Autodesk Inventor part; units mm, degrees
(part 2 of 2)
  arc A140 (-25.4446, 74.7133) -> (-26.798, 74.2336) centre (-25.1834, 71.8276) ccw
  arc A141 (-26.798, 74.2336) -> (-27.2062, 73.5932) centre (-26.3001, 73.4659) ccw
  arc A142 (-21.4794, 73.1947) -> (-22.0085, 74.2336) centre (-22.7699, 73.1916) ccw
  circle A143 centre (-25.9605, 73.338) radius 0.5161
  line L109 (-27.2062, 73.5932) -> (-27.2062, 72.1245)
  line L110 (-27.2062, 72.1245) -> (-24.3395, 72.1245)
  line L111 (-24.3395, 71.7056) -> (-28.3839, 71.7056)
  line L112 (-24.3395, 72.1245) -> (-24.3395, 71.7056)
  line L113 (-21.4733, 70.5884) -> (-21.4794, 73.1947)
  arc A144 (-23.3243, 25.8454) -> (-25.4322, 25.8454) centre (-24.3782, 17.6506) ccw
  arc A145 (-25.4322, 25.8454) -> (-26.7856, 25.3656) centre (-25.171, 22.9597) ccw
  arc A146 (-21.9961, 25.3656) -> (-23.3243, 25.8454) centre (-23.7019, 22.7218) ccw
  arc A147 (-21.4671, 24.3267) -> (-21.9961, 25.3656) centre (-22.7575, 24.3237) ccw
  arc A148 (-26.7856, 25.3656) -> (-27.1938, 24.7252) centre (-26.2877, 24.5979) ccw
  circle A149 centre (-25.9607, 24.5305) radius 0.545
  line L114 (-27.1938, 24.7252) -> (-27.1938, 23.2566)
  line L115 (-27.1938, 23.2566) -> (-24.3272, 23.2566)
  line L116 (-24.3272, 23.2566) -> (-24.3272, 22.8376)
  line L117 (-21.461, 21.7204) -> (-21.4671, 24.3267)
  line L118 (-26.0801, 20.1743) -> (-23.0926, 20.1813)
  arc A150 (-22.5618, 19.8544) -> (-21.3196, 20.5365) centre (-22.5875, 21.3734) ccw
  arc A151 (-23.0926, 20.1813) -> (-21.461, 21.7204) centre (-22.9431, 21.6573) ccw
  line L119 (-22.5618, 19.8544) -> (-25.5493, 19.8474)
  line L120 (-21.0597, 22.9429) -> (-21.0597, 21.4689)
  arc A152 (-21.3196, 20.5365) -> (-21.0597, 21.4689) centre (-22.9439, 21.4916) ccw
  line L121 (-19.9288, 22.9429) -> (-21.0597, 22.9429)
  arc A153 (-18.7198, 21.9341) -> (-19.9288, 22.9429) centre (-20.2582, 21.3193) ccw
  arc A154 (-18.5273, 18.7011) -> (-18.7198, 21.9341) centre (-23.4893, 20.0279) ccw
  arc A155 (-20.2704, 17.1911) -> (-18.5273, 18.7011) centre (-20.3549, 19.0497) ccw
  arc A156 (-25.5493, 19.8474) -> (-27.181, 18.3083) centre (-25.6988, 18.3715) ccw
  arc A157 (-26.0801, 20.1743) -> (-27.3224, 19.4922) centre (-26.0545, 18.6554) ccw
  line L122 (-24.3272, 22.8376) -> (-28.3715, 22.8376)
  arc A158 (-27.3224, 19.4922) -> (-27.5822, 18.5598) centre (-25.698, 18.5371) ccw
  line L123 (-27.5822, 17.0858) -> (-27.5822, 18.5598)
  arc A159 (-28.3715, 22.8376) -> (-30.1146, 21.3277) centre (-28.287, 20.979) ccw
  line L124 (-28.7131, 17.0858) -> (-27.5822, 17.0858)
  arc A160 (-30.1146, 21.3277) -> (-29.9221, 18.0946) centre (-25.1526, 20.0009) ccw
  arc A161 (-29.9221, 18.0946) -> (-28.7131, 17.0858) centre (-28.3837, 18.7095) ccw
  arc A162 (-25.3176, 14.1834) -> (-23.2097, 14.1834) centre (-24.2637, 22.3782) ccw
  arc A163 (-26.6458, 14.6631) -> (-25.3176, 14.1834) centre (-24.94, 17.307) ccw
  arc A164 (-23.2097, 14.1834) -> (-21.8563, 14.6631) centre (-23.4709, 17.0691) ccw
  arc A165 (-21.8563, 14.6631) -> (-21.4481, 15.3035) centre (-22.3542, 15.4308) ccw
  arc A166 (-27.1749, 15.702) -> (-26.6458, 14.6631) centre (-25.8844, 15.705) ccw
  circle A167 centre (-22.6938, 15.5587) radius 0.5161
  line L125 (-21.4481, 15.3035) -> (-21.4481, 16.7721)
  line L126 (-21.4481, 16.7721) -> (-24.3148, 16.7721)
  line L127 (-24.3148, 17.1911) -> (-20.2704, 17.1911)
  line L128 (-24.3148, 16.7721) -> (-24.3148, 17.1911)
  line L129 (-27.181, 18.3083) -> (-27.1749, 15.702)
  arc A168 (-40.1766, 38.6055) -> (-38.0687, 38.6055) centre (-39.1227, 46.8003) ccw
  arc A169 (-38.0687, 38.6055) -> (-36.7153, 39.0853) centre (-38.3299, 41.4912) ccw
  arc A170 (-41.5048, 39.0853) -> (-40.1766, 38.6055) centre (-39.799, 41.7291) ccw
  arc A171 (-42.0338, 40.1242) -> (-41.5048, 39.0853) centre (-40.7434, 40.1272) ccw
  arc A172 (-36.7153, 39.0853) -> (-36.3071, 39.7256) centre (-37.2132, 39.853) ccw
  circle A173 centre (-37.5402, 39.9204) radius 0.545
  line L130 (-36.3071, 39.7256) -> (-36.3071, 41.1943)
  line L131 (-36.3071, 41.1943) -> (-39.1737, 41.1943)
  line L132 (-39.1737, 41.1943) -> (-39.1737, 41.6132)
  line L133 (-42.0399, 42.7305) -> (-42.0338, 40.1242)
  line L134 (-37.4208, 44.2766) -> (-40.4083, 44.2696)
  arc A174 (-40.9391, 44.5964) -> (-42.1813, 43.9143) centre (-40.9134, 43.0775) ccw
  arc A175 (-40.4083, 44.2696) -> (-42.0399, 42.7305) centre (-40.5578, 42.7936) ccw
  line L135 (-40.9391, 44.5964) -> (-37.9516, 44.6034)
  line L136 (-42.4412, 41.508) -> (-42.4412, 42.982)
  arc A176 (-42.1813, 43.9143) -> (-42.4412, 42.982) centre (-40.557, 42.9593) ccw
  line L137 (-43.5721, 41.508) -> (-42.4412, 41.508)
  arc A177 (-44.7811, 42.5167) -> (-43.5721, 41.508) centre (-43.2427, 43.1316) ccw
  arc A178 (-44.9736, 45.7498) -> (-44.7811, 42.5167) centre (-40.0116, 44.423) ccw
  arc A179 (-43.2305, 47.2598) -> (-44.9736, 45.7498) centre (-43.146, 45.4011) ccw
  arc A180 (-37.9516, 44.6034) -> (-36.3199, 46.1426) centre (-37.8021, 46.0794) ccw
  arc A181 (-37.4208, 44.2766) -> (-36.1785, 44.9587) centre (-37.4464, 45.7955) ccw
  line L138 (-39.1737, 41.6132) -> (-35.1294, 41.6132)
  arc A182 (-36.1785, 44.9587) -> (-35.9187, 45.891) centre (-37.8029, 45.9137) ccw
  line L139 (-35.9187, 47.365) -> (-35.9187, 45.891)
  arc A183 (-35.1294, 41.6132) -> (-33.3863, 43.1232) centre (-35.2139, 43.4719) ccw
  line L140 (-34.7877, 47.365) -> (-35.9187, 47.365)
  arc A184 (-33.3863, 43.1232) -> (-33.5788, 46.3563) centre (-38.3483, 44.45) ccw
  arc A185 (-33.5788, 46.3563) -> (-34.7877, 47.365) centre (-35.1172, 45.7414) ccw
  arc A186 (-38.1832, 50.2675) -> (-40.2912, 50.2675) centre (-39.2372, 42.0727) ccw
  arc A187 (-36.8551, 49.7878) -> (-38.1832, 50.2675) centre (-38.5609, 47.1439) ccw
  arc A188 (-40.2912, 50.2675) -> (-41.6446, 49.7878) centre (-40.03, 47.3818) ccw
  arc A189 (-41.6446, 49.7878) -> (-42.0528, 49.1474) centre (-41.1467, 49.02) ccw
  arc A190 (-36.326, 48.7488) -> (-36.8551, 49.7878) centre (-37.6165, 48.7458) ccw
  circle A191 centre (-40.8071, 48.8922) radius 0.5161
  line L141 (-42.0528, 49.1474) -> (-42.0528, 47.6787)
  line L142 (-42.0528, 47.6787) -> (-39.1861, 47.6787)
  line L143 (-39.1861, 47.2598) -> (-43.2305, 47.2598)
  line L144 (-39.1861, 47.6787) -> (-39.1861, 47.2598)
  line L145 (-36.3199, 46.1426) -> (-36.326, 48.7488)
  line L146 (-31.75, 88.9) -> (-31.75, 0) construction
  arc A192 (-25.3307, 38.6055) -> (-23.2228, 38.6055) centre (-24.2767, 46.8003) ccw
  arc A193 (-23.2228, 38.6055) -> (-21.8693, 39.0853) centre (-23.4839, 41.4912) ccw
  arc A194 (-20.2834, 41.6132) -> (-18.5403, 43.1232) centre (-20.3679, 43.4719) ccw
  arc A195 (-21.3326, 44.9587) -> (-21.0728, 45.891) centre (-22.9569, 45.9137) ccw
  arc A196 (-18.5403, 43.1232) -> (-18.7328, 46.3563) centre (-23.5023, 44.45) ccw
  arc A197 (-18.7328, 46.3563) -> (-19.9418, 47.365) centre (-20.2712, 45.7414) ccw
  line L147 (-19.9418, 47.365) -> (-21.0728, 47.365)
  line L148 (-21.0728, 47.365) -> (-21.0728, 45.891)
  line L149 (-22.5749, 44.2766) -> (-25.5624, 44.2696)
  line L150 (-26.0931, 44.5964) -> (-23.1056, 44.6034)
  line L151 (-24.3402, 47.6787) -> (-24.3402, 47.2598)
  line L152 (-24.3402, 47.2598) -> (-28.3846, 47.2598)
  line L153 (-21.474, 46.1426) -> (-21.4801, 48.7488)
  line L154 (-27.2069, 47.6787) -> (-24.3402, 47.6787)
  circle A198 centre (-25.9611, 48.8922) radius 0.5161
  line L155 (-27.2069, 49.1474) -> (-27.2069, 47.6787)
  arc A199 (-26.7987, 49.7878) -> (-27.2069, 49.1474) centre (-26.3007, 49.02) ccw
  arc A200 (-25.4452, 50.2675) -> (-26.7987, 49.7878) centre (-25.1841, 47.3818) ccw
  arc A201 (-23.3373, 50.2675) -> (-25.4452, 50.2675) centre (-24.3913, 42.0727) ccw
  arc A202 (-22.0092, 49.7878) -> (-23.3373, 50.2675) centre (-23.7149, 47.1439) ccw
  arc A203 (-21.4801, 48.7488) -> (-22.0092, 49.7878) centre (-22.7706, 48.7458) ccw
  arc A204 (-21.8693, 39.0853) -> (-21.4611, 39.7256) centre (-22.3673, 39.853) ccw
  circle A205 centre (-22.6942, 39.9204) radius 0.545
  line L156 (-21.4611, 39.7256) -> (-21.4611, 41.1943)
  line L157 (-21.4611, 41.1943) -> (-24.3278, 41.1943)
  line L158 (-24.3278, 41.6132) -> (-20.2834, 41.6132)
  line L159 (-24.3278, 41.1943) -> (-24.3278, 41.6132)
  arc A206 (-22.5749, 44.2766) -> (-21.3326, 44.9587) centre (-22.6005, 45.7955) ccw
  arc A207 (-23.1056, 44.6034) -> (-21.474, 46.1426) centre (-22.9562, 46.0794) ccw
  arc A208 (-26.6588, 39.0853) -> (-25.3307, 38.6055) centre (-24.9531, 41.7291) ccw
  arc A209 (-27.1879, 40.1242) -> (-26.6588, 39.0853) centre (-25.8974, 40.1272) ccw
  line L160 (-27.194, 42.7305) -> (-27.1879, 40.1242)
  arc A210 (-26.0931, 44.5964) -> (-27.3354, 43.9143) centre (-26.0675, 43.0775) ccw
  arc A211 (-25.5624, 44.2696) -> (-27.194, 42.7305) centre (-25.7118, 42.7936) ccw
  line L161 (-27.5952, 41.508) -> (-27.5952, 42.982)
  arc A212 (-27.3354, 43.9143) -> (-27.5952, 42.982) centre (-25.7111, 42.9593) ccw
  arc A213 (-28.3846, 47.2598) -> (-30.1277, 45.7498) centre (-28.3001, 45.4011) ccw
  line L162 (-28.7262, 41.508) -> (-27.5952, 41.508)
  arc A214 (-29.9351, 42.5167) -> (-28.7262, 41.508) centre (-28.3968, 43.1316) ccw
  arc A215 (-30.1277, 45.7498) -> (-29.9351, 42.5167) centre (-25.1657, 44.423) ccw
  line L163 (-39.1737, 68.8958) -> (-24.3278, 44.45) construction
  line L164 (-39.1737, 44.45) -> (-24.3272, 68.8958) construction
  arc A216 (-32.7536, 50.8283) -> (-30.6456, 50.8283) centre (-31.6996, 59.0231) ccw
  arc A217 (-30.6456, 50.8283) -> (-29.2922, 51.308) centre (-30.9068, 53.714) ccw
  arc A218 (-34.0817, 51.308) -> (-32.7536, 50.8283) centre (-32.3759, 53.9519) ccw
  arc A219 (-34.6108, 52.3469) -> (-34.0817, 51.308) centre (-33.3203, 52.3499) ccw
  arc A220 (-29.2922, 51.308) -> (-28.884, 51.9484) centre (-29.7901, 52.0757) ccw
  circle A221 centre (-30.1171, 52.1431) radius 0.545
  line L165 (-28.884, 51.9484) -> (-28.884, 53.417)
  line L166 (-28.884, 53.417) -> (-31.7507, 53.417)
  line L167 (-31.7507, 53.417) -> (-31.7507, 53.836)
  line L168 (-34.6169, 54.9532) -> (-34.6108, 52.3469)
  line L169 (-29.9978, 56.4993) -> (-32.9852, 56.4923)
  arc A222 (-33.516, 56.8192) -> (-34.7583, 56.1371) centre (-33.4904, 55.3003) ccw
  arc A223 (-32.9852, 56.4923) -> (-34.6169, 54.9532) centre (-33.1347, 55.0164) ccw
  line L170 (-33.516, 56.8192) -> (-30.5285, 56.8262)
  line L171 (-35.0181, 53.7307) -> (-35.0181, 55.2047)
  arc A224 (-34.7583, 56.1371) -> (-35.0181, 55.2047) centre (-33.1339, 55.182) ccw
  line L172 (-36.1491, 53.7307) -> (-35.0181, 53.7307)
  arc A225 (-37.358, 54.7395) -> (-36.1491, 53.7307) centre (-35.8197, 55.3544) ccw
  arc A226 (-37.5506, 57.9726) -> (-37.358, 54.7395) centre (-32.5885, 56.6458) ccw
  arc A227 (-35.8074, 59.4825) -> (-37.5506, 57.9726) centre (-35.7229, 57.6239) ccw
  arc A228 (-30.5285, 56.8262) -> (-28.8969, 58.3653) centre (-30.379, 58.3022) ccw
  arc A229 (-29.9978, 56.4993) -> (-28.7555, 57.1814) centre (-30.0234, 58.0183) ccw
  line L173 (-31.7507, 53.836) -> (-27.7063, 53.836)
  arc A230 (-28.7555, 57.1814) -> (-28.4957, 58.1138) centre (-30.3798, 58.1365) ccw
  line L174 (-28.4957, 59.5878) -> (-28.4957, 58.1138)
  arc A231 (-27.7063, 53.836) -> (-25.9632, 55.346) centre (-27.7908, 55.6946) ccw
  line L175 (-27.3647, 59.5878) -> (-28.4957, 59.5878)
  arc A232 (-25.9632, 55.346) -> (-26.1557, 58.579) centre (-30.9252, 56.6728) ccw
  arc A233 (-26.1557, 58.579) -> (-27.3647, 59.5878) centre (-27.6941, 57.9642) ccw
  arc A234 (-30.7602, 62.4903) -> (-32.8681, 62.4903) centre (-31.8141, 54.2955) ccw
  arc A235 (-29.4321, 62.0105) -> (-30.7602, 62.4903) centre (-31.1378, 59.3667) ccw
  arc A236 (-32.8681, 62.4903) -> (-34.2215, 62.0105) centre (-32.607, 59.6046) ccw
  arc A237 (-34.2215, 62.0105) -> (-34.6298, 61.3701) centre (-33.7236, 61.2428) ccw
  arc A238 (-28.903, 60.9716) -> (-29.4321, 62.0105) centre (-30.1934, 60.9686) ccw
  circle A239 centre (-33.384, 61.1149) radius 0.5161
  line L176 (-34.6298, 61.3701) -> (-34.6298, 59.9015)
  line L177 (-34.6298, 59.9015) -> (-31.7631, 59.9015)
  line L178 (-31.7631, 59.4825) -> (-35.8074, 59.4825)
  line L179 (-31.7631, 59.9015) -> (-31.7631, 59.4825)
  line L180 (-28.8969, 58.3653) -> (-28.903, 60.9716)
  line L181 (-50.4381, 84.1079) -> (-54.8347, 75.4711)
  line L182 (-54.8347, 75.4711) -> (-56.2838, 75.4711)
  line L183 (-56.2838, 75.4711) -> (-51.6402, 84.4373)
  line L184 (-51.6402, 84.4373) -> (-56.8849, 84.4373)
  line L185 (-56.8849, 84.4373) -> (-56.8849, 85.6311)
  line L186 (-56.8849, 85.6311) -> (-50.4381, 85.6311)
  line L187 (-50.4381, 85.6311) -> (-50.4381, 84.1079)
  line L188 (-13.0619, 5.1366) -> (-8.6653, 13.7735)
  line L189 (-8.6653, 13.7735) -> (-7.2162, 13.7735)
  line L190 (-7.2162, 13.7735) -> (-11.8598, 4.8073)
  line L191 (-11.8598, 4.8073) -> (-6.6151, 4.8073)
  line L192 (-6.6151, 4.8073) -> (-6.6151, 3.6135)
  line L193 (-6.6151, 3.6135) -> (-13.0619, 3.6135)
  line L194 (-13.0619, 3.6135) -> (-13.0619, 5.1366)
  line L195 (-50.4381, 84.1079) -> (-54.8347, 75.4711)
  line L196 (-54.8347, 75.4711) -> (-56.2838, 75.4711)
  line L197 (-56.2838, 75.4711) -> (-51.6402, 84.4373)
  line L198 (-51.6402, 84.4373) -> (-56.8849, 84.4373)
  line L199 (-56.8849, 84.4373) -> (-56.8849, 85.6311)
  line L200 (-56.8849, 85.6311) -> (-50.4381, 85.6311)
  line L201 (-50.4381, 85.6311) -> (-50.4381, 84.1079)
  line L202 (-13.0619, 5.1366) -> (-8.6653, 13.7735)
  line L203 (-8.6653, 13.7735) -> (-7.2162, 13.7735)
  line L204 (-7.2162, 13.7735) -> (-11.8598, 4.8073)
  line L205 (-11.8598, 4.8073) -> (-6.6151, 4.8073)
  line L206 (-6.6151, 4.8073) -> (-6.6151, 3.6135)
  line L207 (-6.6151, 3.6135) -> (-13.0619, 3.6135)
  line L208 (-13.0619, 3.6135) -> (-13.0619, 5.1366)
  point P0 (-39.1737, 20.0009)
  point P1 (-53.7479, 68.8958)
  point P2 (-9.7521, 20.0042)
  point P3 (-13.4723, 102.9238)
  point P4 (-39.1737, 20.0009)
  point P5 (-53.7479, 68.8958)
  point P6 (-9.7521, 20.0042)
  point P7 (-24.3263, 68.8958)
  point P8 (-24.3272, 20.0009)
  point P9 (-24.3272, 20.0009)
  point P10 (-39.1737, 44.45)
  point P11 (-24.3263, 44.45)
  point P12 (-24.3278, 44.45)
  point P13 (-24.3278, 44.45)
  point P14 (-24.3278, 44.45)
  point P15 (-31.7504, 56.6729)
  point P16 (-31.7507, 56.6728)
  point P17 (-31.7507, 56.6728)
  dimension "d103" = 8.4153
  dimension "d105" = 0.508
  dimension "d106" = 0.508
  constraints: 440 point on circle, 336 end point, 240 centre point, 40 perpendicular, 40 tangent, 16 vertical, 8 horizontal, 3 midpoint, 1 parallel, 1 symmetric about line, 5 other
  measures "d103" distance of L12.end L14.start
  measures "d105" distance between parallel lines of L15 L7
  measures "d106" distance between parallel lines of L16 L11
extrude "Extrusion20" add sketch "Sketch17" along normal blind 0.4 contours A112 L95 L96 A116 A117 A115 L93 L2 | L2 L93 L89 L91 L94 A111 A110 A108 A114 A109 L90 A107 L92 A113 A112 | L193 L194 L188 L189 L2 L190 L191 | L2 L191 L192 L193 | L189 L190 L2 | L40 A34 A33 A32 L39 L38 L37 L36 A31 A30 A29 A28 A27 L35 A26 L34 A25 A24 L33 | L56 A58 A57 A56 L55 L54 L53 L52 A55 A54 A53 A52 A51 L51 A50 L50 A49 A48 L49 | L72 A82 A81 A80 L71 L70 L69 L68 A79 A78 A77 A76 A75 L67 A74 L66 A73 A72 L65 | A122 A123 L101 A127 L102 A133 A134 L107 L108 A137 A136 A135 L106 L100 L99 L98 A124 A121 A120 | A150 A152 L120 L121 A153 A154 A155 L127 L128 L126 L125 A165 A164 A162 A163 A166 L129 A156 L119 | A174 A176 L136 L137 A177 A178 A179 L143 L144 L142 L141 A189 A188 A186 A187 A190 L145 A180 L135 | A210 A212 L161 L162 A214 A215 A213 L152 L151 L154 L155 A199 A200 A201 A202 A203 L153 A207 L150 | A222 A224 L171 L172 A225 A226 A227 L178 L179 L177 L176 A237 A236 A234 A235 A238 L180 A228 L170 | L181 L182 L183 L184 L185 L186 L187 bodies 1
sketch "Sketch18" plane through (0, 0, -0.2) normal (0, 0, -1) x (-1, 0, 0)
  line L0 (0, 0) -> (-63.5, 0)
  line L1 (-63.5, 0) -> (-63.5, 88.9)
  line L2 (-63.5, 88.9) -> (0, 88.9)
  line L3 (0, 88.9) -> (0, 0)
  constraints: 8 end point, 2 parallel, 1 horizontal, 1 perpendicular
extrude "Extrusion21" add sketch "Sketch18" along normal blind 0.4 bodies 3
fillet "Fillet2" radius 3.175 8 edges at (63.5, 0, 0.2) (63.5, 88.9, 0.2) (0, 0, 0.2) (0, 88.9, 0.2) (63.5, 0, -0.3) (63.5, 88.9, -0.3) (0, 0, -0.3) (0, 88.9, -0.3)
extrude "Extrusion22" cut sketch "Sketch17" along normal blind 0.4 contours A112 L95 L96 A116 A117 A115 L93 L2 | L2 L93 L89 L91 L94 A111 A110 A108 A114 A109 L90 A107 L92 A113 A112 | L193 L194 L188 L189 L2 L190 L191 | L2 L191 L192 L193 | L189 L190 L2 | L40 A34 A33 A32 L39 L38 L37 L36 A31 A30 A29 A28 A27 L35 A26 L34 A25 A24 L33 | L44 A41 A40 L47 L48 A44 A45 A43 L45 L41 L43 L46 A39 A38 A36 A42 A37 L42 A35 | L56 A58 A57 A56 L55 L54 L53 L52 A55 A54 A53 A52 A51 L51 A50 L50 A49 A48 L49 | L60 A65 A64 L63 L64 A68 A69 A67 L61 L57 L59 L62 A63 A62 A60 A66 A61 L58 A59 | L72 A82 A81 A80 L71 L70 L69 L68 A79 A78 A77 A76 A75 L67 A74 L66 A73 A72 L65 | L76 A89 A88 L79 L80 A92 A93 A91 L77 L73 L75 L78 A87 A86 A84 A90 A85 L74 A83 | L88 A106 A105 A104 L87 L86 L85 L84 A103 A102 A101 A100 A99 L83 A98 L82 A97 A96 L81 | A122 A123 L101 A127 L102 A133 A134 L107 L108 A137 A136 A135 L106 L100 L99 L98 A124 A121 A120 | A126 A128 L104 L105 A129 A130 A131 L111 L112 L110 L109 A141 A140 A138 A139 A142 L113 A132 L103 | A146 A147 L117 A151 L118 A157 A158 L123 L124 A161 A160 A159 L122 L116 L115 L114 A148 A145 A144 | A150 A152 L120 L121 A153 A154 A155 L127 L128 L126 L125 A165 A164 A162 A163 A166 L129 A156 L119 | A170 A171 L133 A175 L134 A181 A182 L139 L140 A185 A184 A183 L138 L132 L131 L130 A172 A169 A168 | A174 A176 L136 L137 A177 A178 A179 L143 L144 L142 L141 A189 A188 A186 A187 A190 L145 A180 L135 | A208 A209 L160 A211 L149 A206 A195 L148 L147 A197 A196 A194 L158 L159 L157 L156 A204 A193 A192 | A210 A212 L161 L162 A214 A215 A213 L152 L151 L154 L155 A199 A200 A201 A202 A203 L153 A207 L150 | A218 A219 L168 A223 L169 A229 A230 L174 L175 A233 A232 A231 L173 L167 L166 L165 A220 A217 A216 | A222 A224 L171 L172 A225 A226 A227 L178 L179 L177 L176 A237 A236 A234 A235 A238 L180 A228 L170 | L181 L182 L183 L184 L185 L186 L187 bodies 3
extrude "Extrusion23" add sketch "Sketch17" along normal blind 0.4 contours L44 A41 A40 L47 L48 A44 A45 A43 L45 L41 L43 L46 A39 A38 A36 A42 A37 L42 A35 | L60 A65 A64 L63 L64 A68 A69 A67 L61 L57 L59 L62 A63 A62 A60 A66 A61 L58 A59 | L76 A89 A88 L79 L80 A92 A93 A91 L77 L73 L75 L78 A87 A86 A84 A90 A85 L74 A83 | L88 A106 A105 A104 L87 L86 L85 L84 A103 A102 A101 A100 A99 L83 A98 L82 A97 A96 L81 | A126 A128 L104 L105 A129 A130 A131 L111 L112 L110 L109 A141 A140 A138 A139 A142 L113 A132 L103 | A146 A147 L117 A151 L118 A157 A158 L123 L124 A161 A160 A159 L122 L116 L115 L114 A148 A145 A144 | A170 A171 L133 A175 L134 A181 A182 L139 L140 A185 A184 A183 L138 L132 L131 L130 A172 A169 A168 | A208 A209 L160 A211 L149 A206 A195 L148 L147 A197 A196 A194 L158 L159 L157 L156 A204 A193 A192 | A218 A219 L168 A223 L169 A229 A230 L174 L175 A233 A232 A231 L173 L167 L166 L165 A220 A217 A216 bodies 4
